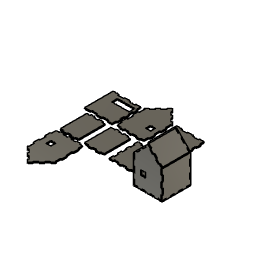
Verkefni2 v12 (Autodesk Fusion 360 design; units mm, degrees)
Autodesk Fusion 360 part; units mm, degrees
sketch "Botnplata Sketch" plane through (0, 0, 0) normal (0, 0, 1) x (1, 0, 0)
  line L0 (0, 0) -> (100, 0)
  line L1 (100, 0) -> (100, 100)
  line L2 (100, 100) -> (0, 100)
  line L3 (0, 100) -> (0, 0)
  dimension "d6" = 100
  dimension "d7" = 100
  constraint horizontal L0
  constraint vertical L1
  constraint horizontal L2
  constraint vertical L3
  constraint coincident L0.start L3.end
  measures "d6" distance of L0.start L2.end
  measures "d7" distance of L0.start L0.end
extrude "Extrude1" add sketch "Botnplata Sketch" along normal blind 4 makes body 1
sketch "Botnplatafingur Sketch" plane through (0, 0, 0) normal (0, -1, 0) x (1, 0, 0)
  line L0 (0, 0) -> (100, 0)
  line L1 (100, 0) -> (100, 4)
  line L2 (100, 4) -> (0, 4)
  line L3 (0, 4) -> (0, 0)
  line L4 (14.2857, 0) -> (28.5714, 0)
  line L5 (28.5714, 0) -> (28.5714, 4)
  line L6 (28.5714, 4) -> (14.2857, 4)
  line L7 (14.2857, 4) -> (14.2857, 0)
  dimension "d13" = 14.2857
  dimension "d14" = 14.2857
  constraint horizontal L4
  constraint vertical L5
  constraint horizontal L6
  constraint vertical L7
  constraint coincident L2 L5.end
  constraint coincident L0 L4.start
  measures "d13" distance of L5.end L6.end
  measures "d14" distance of L3 L7
extrude "Extrude2" cut sketch "Botnplatafingur Sketch" against normal blind 4 contours L0 L2 L4 L5 L6 L7 bodies 1
pattern_linear "R-Pattern1" count 3 spacing 28.5714 along (1, 0, 0) of "Extrude2"
sketch "Sketch3" plane through (100, 0, 0) normal (1, 0, 0) x (0, 1, 0)
  line L0 (0, 0) -> (100, 0)
  line L1 (100, 0) -> (100, 4)
  line L2 (100, 4) -> (0, 4)
  line L3 (0, 4) -> (0, 0)
  line L4 (14.2857, 0) -> (28.5714, 0)
  line L5 (28.5714, 0) -> (28.5714, 4)
  line L6 (28.5714, 4) -> (14.2857, 4)
  line L7 (14.2857, 4) -> (14.2857, 0)
  dimension "d21" = 14.2857
  dimension "d22" = 14.2857
  constraint horizontal L4
  constraint vertical L5
  constraint horizontal L6
  constraint vertical L7
  constraint coincident L2 L5.end
  constraint coincident L0 L4.start
  measures "d21" distance of L5.end L6.end
  measures "d22" distance of L3 L7
extrude "Extrude3" cut sketch "Sketch3" against normal blind 4 contours L0 L2 L4 L5 L6 L7 bodies 1
pattern_linear "R-Pattern2" count 3 spacing 28.5714 along (0, 1, 0) of "Extrude3"
sketch "Botnplafafingur Aftur Sketch" plane through (0, 0, 0) normal (-1, 0, 0) x (0, -1, 0)
  line L0 (-100, 0) -> (0, 0)
  line L1 (0, 0) -> (0, 4)
  line L2 (0, 4) -> (-100, 4)
  line L3 (-100, 4) -> (-100, 0)
  line L4 (-85.7143, 0) -> (-71.4286, 0)
  line L5 (-71.4286, 0) -> (-71.4286, 4)
  line L6 (-71.4286, 4) -> (-85.7143, 4)
  line L7 (-85.7143, 4) -> (-85.7143, 0)
  dimension "d29" = 14.2857
  dimension "d30" = 14.2857
  constraint horizontal L4
  constraint vertical L5
  constraint horizontal L6
  constraint vertical L7
  constraint coincident L2 L5.end
  constraint coincident L0 L4.start
  measures "d29" distance of L5.end L6.end
  measures "d30" distance of L3 L7
extrude "Extrude4" cut sketch "Botnplafafingur Aftur Sketch" against normal blind 4 contours L0 L2 L4 L5 L6 L7 bodies 1
pattern_linear "R-Pattern3" count 3 spacing 28.5714 along (0, -1, 0) of "Extrude4"
sketch "Sketch5" plane through (0, 100, 0) normal (0, 1, 0) x (-1, 0, 0)
  line L0 (-100, 0) -> (0, 0)
  line L1 (0, 0) -> (0, 4)
  line L2 (0, 4) -> (-100, 4)
  line L3 (-100, 4) -> (-100, 0)
  line L4 (-85.7143, 0) -> (-71.4286, 0)
  line L5 (-71.4286, 0) -> (-71.4286, 4)
  line L6 (-71.4286, 4) -> (-85.7143, 4)
  line L7 (-85.7143, 4) -> (-85.7143, 0)
  dimension "d37" = 14.2857
  dimension "d38" = 14.2857
  constraint horizontal L4
  constraint vertical L5
  constraint horizontal L6
  constraint vertical L7
  constraint coincident L2 L5.end
  constraint coincident L0 L4.start
  measures "d37" distance of L5.end L6.end
  measures "d38" distance of L3 L7
extrude "Extrude5" cut sketch "Sketch5" against normal blind 4 contours L0 L2 L4 L5 L6 L7 bodies 1
pattern_linear "R-Pattern4" count 3 spacing 28.5714 along (-1, 0, 0) of "Extrude5"
sketch "Sketch6" plane through (0, 0, 0) normal (1, 0, 0) x (0, 1, 0)
  line L0 (0, 0) -> (100, 0)
  line L1 (100, 0) -> (100, 100)
  line L2 (100, 100) -> (0, 100)
  line L3 (0, 100) -> (0, 0)
  dimension "d45" = 100
  dimension "d46" = 100
  constraint horizontal L0
  constraint vertical L1
  constraint horizontal L2
  constraint vertical L3
  constraint coincident L0.start L3.end
  measures "d45" distance of L0.start L2.end
  measures "d46" distance of L0.start L0.end
extrude "Extrude6" add sketch "Sketch6" along normal blind 4 separate body makes body 2
combine "Combine1" operation cut target body 2 tool bodies 1 keep tools
extrude "Extrude7" add 1 faces at (0, 47.619, 68) along direction (-1, 0, 0) blind 4 from surface at -100 separate body on bodies 2 makes body 3
sketch "Sketch9" plane through (0, 0, 0) normal (0, 1, 0) x (1, 0, 0)
  line L0 (0, 0) -> (0, -100)
  line L1 (0, -100) -> (50, -150)
  line L2 (50, -150) -> (100, -100)
  line L3 (100, -100) -> (100, 0)
  line L4 (100, 0) -> (0, 0)
  dimension "d66" = 135
  dimension "d67" = 135
  dimension "d68" = 100
  dimension "d69" = 100
  dimension "d70" = 100
  constraint coincident L0.start L4.end
  constraint vertical L0
  constraint parallel L0 L3
  constraint perpendicular L3 L4
  measures "d66" angle of L0 L1
  measures "d67" angle of L2 L3
  measures "d68" distance of L0.start L0.end
  measures "d69" distance of L2.end L3.end
  measures "d70" distance of L3.end L0.start
extrude "Extrude11" add sketch "Sketch9" along normal blind 4 separate body makes body 4
extrude "Extrude13" add 1 faces at (66.6667, 4, 66.6667) along direction (0, 1, 0) blind 4 from surface at 92 separate body on bodies 4 makes body 5
sketch "Sketch11" plane through (0, 100, 0) normal (0, 1, 0) x (-1, 0, 0)
  line L0 (0, 4) -> (0, 100)
  line L1 (0, 100) -> (-4, 100)
  line L2 (-4, 100) -> (-4, 4)
  line L3 (0, 80) -> (-4, 80)
  line L4 (-4, 80) -> (-4, 60)
  line L5 (-4, 60) -> (0, 60)
  line L6 (0, 60) -> (0, 80)
  line L7 (-4, 4) -> (0, 4)
  dimension "d90" = 20
  dimension "d91" = 20
  constraint horizontal L3
  constraint vertical L4
  constraint horizontal L5
  constraint vertical L6
  constraint coincident L2 L4.end
  constraint coincident L0 L3.start
  measures "d90" distance of L3.start L5.end
  measures "d91" distance of L1 L3
extrude "Extrude15" cut sketch "Sketch11" against normal blind 4 contours L0 L2 L3 L4 L5 L6 bodies 2
pattern_linear "R-Pattern5" count 2 spacing 40 along (0, 0, -1) of "Extrude15"
sketch "Sketch12" plane through (0, 100, 0) normal (0, 1, 0) x (-1, 0, 0)
  line L0 (-100, 100) -> (-100, 4)
  line L1 (-96, 4) -> (-96, 100)
  line L2 (-96, 100) -> (-100, 100)
  line L3 (-96, 80) -> (-100, 80)
  line L4 (-100, 80) -> (-100, 60)
  line L5 (-100, 60) -> (-96, 60)
  line L6 (-96, 60) -> (-96, 80)
  line L7 (-100, 4) -> (-96, 4)
  dimension "d98" = 20
  dimension "d99" = 20
  constraint horizontal L3
  constraint vertical L4
  constraint horizontal L5
  constraint vertical L6
  constraint coincident L0 L4.end
  constraint coincident L1 L3.start
  measures "d98" distance of L3.start L5.end
  measures "d99" distance of L2 L3
extrude "Extrude16" cut sketch "Sketch12" against normal blind 4 contours L0 L1 L3 L4 L5 L6 bodies 3
pattern_linear "R-Pattern6" count 2 spacing 40 along (0, 0, -1) of "Extrude16"
sketch "Sketch13" plane through (0, 0, 0) normal (0, -1, 0) x (1, 0, 0)
  line L0 (0, 4) -> (4, 4)
  line L1 (4, 4) -> (4, 100)
  line L2 (4, 100) -> (0, 100)
  line L3 (0, 100) -> (0, 4)
  line L4 (0, 80) -> (4, 80)
  line L5 (4, 80) -> (4, 60)
  line L6 (4, 60) -> (0, 60)
  line L7 (0, 60) -> (0, 80)
  dimension "d106" = 20
  dimension "d107" = 20
  constraint horizontal L4
  constraint vertical L5
  constraint horizontal L6
  constraint vertical L7
  constraint coincident L1 L5.end
  constraint coincident L3 L4.start
  measures "d106" distance of L2 L4
  measures "d107" distance of L4.start L6.end
extrude "Extrude17" cut sketch "Sketch13" against normal blind 4 contours L1 L3 L4 L5 L6 L7 bodies 2
pattern_linear "R-Pattern7" count 2 spacing 40 along (0, 0, -1) of "Extrude17"
sketch "Sketch14" plane through (0, 0, 0) normal (0, -1, 0) x (1, 0, 0)
  line L0 (100, 4) -> (100, 100)
  line L1 (100, 100) -> (96, 100)
  line L2 (96, 100) -> (96, 4)
  line L3 (96, 80) -> (100, 80)
  line L4 (100, 80) -> (100, 60)
  line L5 (100, 60) -> (96, 60)
  line L6 (96, 60) -> (96, 80)
  line L7 (96, 4) -> (100, 4)
  dimension "d114" = 20
  dimension "d115" = 20
  constraint horizontal L3
  constraint vertical L4
  constraint horizontal L5
  constraint vertical L6
  constraint coincident L0 L4.end
  constraint coincident L2 L3.start
  measures "d114" distance of L3.end L4.end
  measures "d115" distance of L1 L3
extrude "Extrude18" cut sketch "Sketch14" against normal blind 4 contours L0 L2 L3 L4 L5 L6 bodies 3
pattern_linear "R-Pattern8" count 2 spacing 40 along (0, 0, -1) of "Extrude18"
combine "Combine3" operation cut target body 4 tool bodies 2 1 3 keep tools
combine "Combine4" operation cut target body 5 tool bodies 2 1 3 keep tools
sketch "Sketch25" plane through (100, 0, 100) normal (0.707107, 0, 0.707107) x (0, 1, 0)
  line L0 (96, 0) -> (100, 0)
  line L1 (100, 0) -> (100, 70.7107)
  line L2 (100, 70.7107) -> (96, 70.7107)
  line L3 (100, 70.7107) -> (0, 70.7107)
  line L4 (0, 70.7107) -> (0, 3)
  line L5 (0, 3) -> (100, 3)
  line L6 (100, 3) -> (100, 70.7107)
  dimension "d123" = 100
  dimension "d136" = 67.7107
  constraint horizontal L3
  constraint vertical L4
  constraint horizontal L5
  constraint vertical L6
  constraint coincident L1.end L2.start
  measures "d123" distance of L4.end L5.end
  measures "d136" distance of L3.end L4.end
extrude "Extrude19" add sketch "Sketch25" against normal blind 4 separate body makes body 6
sketch "Sketch26" plane through (100, 0, 100) normal (0.707107, 0, 0.707107) x (0, 1, 0)
  line L0 (0, 70.7107) -> (0, 0)
  line L1 (0, 0) -> (4, 0)
  line L2 (4, 0) -> (4, 70.7107)
  line L3 (4, 70.7107) -> (0, 70.7107)
  line L4 (0, 56.5685) -> (4, 56.5685)
  line L5 (4, 56.5685) -> (4, 42.4264)
  line L6 (4, 42.4264) -> (0, 42.4264)
  line L7 (0, 42.4264) -> (0, 56.5685)
  dimension "d126" = 14.1421
  dimension "d127" = 14.1421
  constraint horizontal L4
  constraint vertical L5
  constraint horizontal L6
  constraint vertical L7
  constraint coincident L2 L5.end
  constraint coincident L0 L4.start
  measures "d126" distance of L4.end L5.end
  measures "d127" distance of L3 L4
extrude "Extrude20" cut sketch "Sketch26" against normal blind 4 contours L0 L2 L4 L5 L6 L7 bodies 4
pattern_linear "R-Pattern9" count 2 spacing 28.2843 along (0.707107, 0, -0.707107) of "Extrude20"
sketch "Sketch27" plane through (100, 0, 100) normal (0.707107, 0, 0.707107) x (0, 1, 0)
  line L0 (96, 70.7107) -> (96, 0)
  line L1 (96, 0) -> (100, 0)
  line L2 (100, 0) -> (100, 70.7107)
  line L3 (100, 70.7107) -> (96, 70.7107)
  line L4 (96, 56.5685) -> (100, 56.5685)
  line L5 (100, 56.5685) -> (100, 42.4264)
  line L6 (100, 42.4264) -> (96, 42.4264)
  line L7 (96, 42.4264) -> (96, 56.5685)
  dimension "d137" = 14.1421
  dimension "d138" = 14.1421
  constraint horizontal L4
  constraint vertical L5
  constraint horizontal L6
  constraint vertical L7
  constraint coincident L2 L5.end
  constraint coincident L0 L4.start
  measures "d137" distance of L4.end L5.end
  measures "d138" distance of L3 L4
extrude "Extrude21" cut sketch "Sketch27" against normal blind 4 contours L0 L2 L4 L5 L6 L7 bodies 5
pattern_linear "R-Pattern10" count 2 spacing 28.2843 along (0.707107, 0, -0.707107) of "Extrude21"
sketch "Sketch28" plane through (-50, 0, 50) normal (-0.707107, 0, 0.707107) x (0, -1, 0)
  line L0 (0, 70.7107) -> (0, 141.4214)
  line L1 (0, 141.4214) -> (-4, 141.4214)
  line L2 (-4, 141.4214) -> (-4, 70.7107)
  line L3 (-4, 70.7107) -> (0, 70.7107)
  line L4 (-4, 127.2792) -> (0, 127.2792)
  line L5 (0, 127.2792) -> (0, 113.1371)
  line L6 (0, 113.1371) -> (-4, 113.1371)
  line L7 (-4, 113.1371) -> (-4, 127.2792)
  dimension "d145" = 14.1421
  dimension "d146" = 14.1421
  constraint horizontal L4
  constraint vertical L5
  constraint horizontal L6
  constraint vertical L7
  constraint coincident L0 L5.end
  constraint coincident L2 L4.start
  measures "d145" distance of L4.end L5.end
  measures "d146" distance of L1 L4
extrude "Extrude22" cut sketch "Sketch28" against normal blind 4 contours L0 L2 L4 L5 L6 L7 bodies 4
pattern_linear "R-Pattern11" count 2 spacing 28.2843 along (-0.707107, 0, -0.707107) of "Extrude22"
sketch "Sketch29" plane through (-50, 0, 50) normal (-0.707107, 0, 0.707107) x (0, -1, 0)
  line L0 (-96, 70.7107) -> (-96, 141.4214)
  line L1 (-96, 141.4214) -> (-100, 141.4214)
  line L2 (-100, 141.4214) -> (-100, 70.7107)
  line L3 (-100, 70.7107) -> (-96, 70.7107)
  line L4 (-100, 127.2792) -> (-96, 127.2792)
  line L5 (-96, 127.2792) -> (-96, 113.1371)
  line L6 (-96, 113.1371) -> (-100, 113.1371)
  line L7 (-100, 113.1371) -> (-100, 127.2792)
  dimension "d153" = 14.1421
  dimension "d154" = 14.1421
  constraint horizontal L4
  constraint vertical L5
  constraint horizontal L6
  constraint vertical L7
  constraint coincident L0 L5.end
  constraint coincident L2 L4.start
  measures "d153" distance of L4.end L5.end
  measures "d154" distance of L1 L4
extrude "Extrude23" cut sketch "Sketch29" against normal blind 4 contours L0 L2 L4 L5 L6 L7 bodies 5
pattern_linear "R-Pattern12" count 2 spacing 28.2843 along (-0.707107, 0, -0.707107) of "Extrude23"
combine "Combine5" operation cut target body 6 tool bodies 5 4 keep tools
sketch "Sketch30" plane through (0, 100, 0) normal (0, 1, 0) x (-1, 0, 0)
  line L0 (-22.8284, 117.1716) -> (-20, 120)
  line L1 (-20, 120) -> (-30, 130)
  line L2 (-30, 130) -> (-32.8284, 127.1716)
  line L3 (-32.8284, 127.1716) -> (-42.8284, 137.1716)
  line L4 (-42.8284, 137.1716) -> (-40, 140)
  line L5 (-40, 140) -> (-50, 150)
  line L6 (-50, 150) -> (-60, 140)
  line L7 (-60, 140) -> (-57.1716, 137.1716)
  line L8 (-57.1716, 137.1716) -> (-67.1716, 127.1716)
  line L9 (-67.1716, 127.1716) -> (-70, 130)
  line L10 (-70, 130) -> (-80, 120)
  line L11 (-80, 120) -> (-77.1716, 117.1716)
  line L12 (-77.1716, 117.1716) -> (-87.1716, 107.1716)
  line L13 (-87.1716, 107.1716) -> (-90, 110)
  line L14 (-90, 110) -> (-100, 100)
  line L15 (-100, 100) -> (-96, 100)
  line L16 (-96, 100) -> (-96, 80)
  line L17 (-96, 80) -> (-100, 80)
  line L18 (-100, 80) -> (-100, 60)
  line L19 (-100, 60) -> (-96, 60)
  line L20 (-96, 60) -> (-96, 40)
  line L21 (-96, 40) -> (-100, 40)
  line L22 (-100, 40) -> (-100, 20)
  line L23 (-100, 20) -> (-96, 20)
  line L24 (-96, 20) -> (-96, 4)
  line L25 (-96, 4) -> (-85.7143, 4)
  line L26 (-85.7143, 4) -> (-85.7143, 0)
  line L27 (-85.7143, 0) -> (-71.4286, 0)
  line L28 (-71.4286, 0) -> (-71.4286, 4)
  line L29 (-71.4286, 4) -> (-57.1429, 4)
  line L30 (-57.1429, 4) -> (-57.1429, 0)
  line L31 (-57.1429, 0) -> (-42.8571, 0)
  line L32 (-42.8571, 0) -> (-42.8571, 4)
  line L33 (-42.8571, 4) -> (-28.5714, 4)
  line L34 (-28.5714, 4) -> (-28.5714, 0)
  line L35 (-28.5714, 0) -> (-14.2857, 0)
  line L36 (-14.2857, 0) -> (-14.2857, 4)
  line L37 (-14.2857, 4) -> (-4, 4)
  line L38 (-4, 4) -> (-4, 20)
  line L39 (-4, 20) -> (0, 20)
  line L40 (0, 20) -> (0, 40)
  line L41 (0, 40) -> (-4, 40)
  line L42 (-4, 40) -> (-4, 60)
  line L43 (-4, 60) -> (0, 60)
  line L44 (0, 60) -> (0, 80)
  line L45 (0, 80) -> (-4, 80)
  line L46 (-4, 80) -> (-4, 100)
  line L47 (-4, 100) -> (0, 100)
  line L48 (0, 100) -> (-10, 110)
  line L49 (-10, 110) -> (-12.8284, 107.1716)
  line L50 (-12.8284, 107.1716) -> (-22.8284, 117.1716)
  line L51 (-80, 60) -> (-63.3333, 60)
  line L52 (-63.3333, 60) -> (-63.3333, 43.3333)
  line L53 (-63.3333, 43.3333) -> (-80, 43.3333)
  line L54 (-80, 43.3333) -> (-80, 60)
  dimension "d165" = 16.6667
  dimension "d166" = 16.6667
  constraint horizontal L51
  constraint vertical L52
  constraint horizontal L53
  constraint vertical L54
  measures "d165" distance of L51.start L53.end
  measures "d166" distance of L51.start L51.end
extrude "Extrude24" cut sketch "Sketch30" against normal blind 4 contours L51 L52 L53 L54 bodies 5
sketch "Sketch31" plane through (0, 0, 0) normal (-1, 0, 0) x (0, -1, 0)
  line L0 (-4, 40) -> (0, 40)
  line L1 (0, 40) -> (0, 60)
  line L2 (0, 60) -> (-4, 60)
  line L3 (-4, 60) -> (-4, 80)
  line L4 (-4, 80) -> (0, 80)
  line L5 (0, 80) -> (0, 100)
  line L6 (0, 100) -> (-100, 100)
  line L7 (-100, 100) -> (-100, 80)
  line L8 (-100, 80) -> (-96, 80)
  line L9 (-96, 80) -> (-96, 60)
  line L10 (-96, 60) -> (-100, 60)
  line L11 (-100, 60) -> (-100, 40)
  line L12 (-100, 40) -> (-96, 40)
  line L13 (-96, 40) -> (-96, 20)
  line L14 (-96, 20) -> (-100, 20)
  line L15 (-100, 20) -> (-100, 4)
  line L16 (-100, 4) -> (-85.7143, 4)
  line L17 (-85.7143, 4) -> (-85.7143, 0)
  line L18 (-85.7143, 0) -> (-71.4286, 0)
  line L19 (-71.4286, 0) -> (-71.4286, 4)
  line L20 (-71.4286, 4) -> (-57.1429, 4)
  line L21 (-57.1429, 4) -> (-57.1429, 0)
  line L22 (-57.1429, 0) -> (-42.8571, 0)
  line L23 (-42.8571, 0) -> (-42.8571, 4)
  line L24 (-42.8571, 4) -> (-28.5714, 4)
  line L25 (-28.5714, 4) -> (-28.5714, 0)
  line L26 (-28.5714, 0) -> (-14.2857, 0)
  line L27 (-14.2857, 0) -> (-14.2857, 4)
  line L28 (-14.2857, 4) -> (0, 4)
  line L29 (0, 4) -> (0, 20)
  line L30 (0, 20) -> (-4, 20)
  line L31 (-4, 20) -> (-4, 40)
  line L32 (-85, 10) -> (-65, 10)
  line L33 (-65, 10) -> (-65, 70)
  line L34 (-65, 70) -> (-85, 70)
  line L35 (-85, 70) -> (-85, 10)
  dimension "d169" = 60
  dimension "d170" = 20
  constraint horizontal L32
  constraint vertical L33
  constraint horizontal L34
  constraint vertical L35
  measures "d169" distance of L32.start L34.end
  measures "d170" distance of L32.start L32.end
extrude "Extrude25" cut sketch "Sketch31" against normal blind 4 contours L32 L33 L34 L35 bodies 2
sketch "Sketch32" plane through (0, 0, 0) normal (0, -1, 0) x (1, 0, 0)
  line L0 (20, 120) -> (22.8284, 117.1716)
  line L1 (22.8284, 117.1716) -> (12.8284, 107.1716)
  line L2 (12.8284, 107.1716) -> (10, 110)
  line L3 (10, 110) -> (0, 100)
  line L4 (0, 100) -> (4, 100)
  line L5 (4, 100) -> (4, 80)
  line L6 (4, 80) -> (0, 80)
  line L7 (0, 80) -> (0, 60)
  line L8 (0, 60) -> (4, 60)
  line L9 (4, 60) -> (4, 40)
  line L10 (4, 40) -> (0, 40)
  line L11 (0, 40) -> (0, 20)
  line L12 (0, 20) -> (4, 20)
  line L13 (4, 20) -> (4, 4)
  line L14 (4, 4) -> (14.2857, 4)
  line L15 (14.2857, 4) -> (14.2857, 0)
  line L16 (14.2857, 0) -> (28.5714, 0)
  line L17 (28.5714, 0) -> (28.5714, 4)
  line L18 (28.5714, 4) -> (42.8571, 4)
  line L19 (42.8571, 4) -> (42.8571, 0)
  line L20 (42.8571, 0) -> (57.1429, 0)
  line L21 (57.1429, 0) -> (57.1429, 4)
  line L22 (57.1429, 4) -> (71.4286, 4)
  line L23 (71.4286, 4) -> (71.4286, 0)
  line L24 (71.4286, 0) -> (85.7143, 0)
  line L25 (85.7143, 0) -> (85.7143, 4)
  line L26 (85.7143, 4) -> (96, 4)
  line L27 (96, 4) -> (96, 20)
  line L28 (96, 20) -> (100, 20)
  line L29 (100, 20) -> (100, 40)
  line L30 (100, 40) -> (96, 40)
  line L31 (96, 40) -> (96, 60)
  line L32 (96, 60) -> (100, 60)
  line L33 (100, 60) -> (100, 80)
  line L34 (100, 80) -> (96, 80)
  line L35 (96, 80) -> (96, 100)
  line L36 (96, 100) -> (100, 100)
  line L37 (100, 100) -> (90, 110)
  line L38 (90, 110) -> (87.1716, 107.1716)
  line L39 (87.1716, 107.1716) -> (77.1716, 117.1716)
  line L40 (77.1716, 117.1716) -> (80, 120)
  line L41 (80, 120) -> (70, 130)
  line L42 (70, 130) -> (67.1716, 127.1716)
  line L43 (67.1716, 127.1716) -> (57.1716, 137.1716)
  line L44 (57.1716, 137.1716) -> (60, 140)
  line L45 (60, 140) -> (50, 150)
  line L46 (50, 150) -> (40, 140)
  line L47 (40, 140) -> (42.8284, 137.1716)
  line L48 (42.8284, 137.1716) -> (32.8284, 127.1716)
  line L49 (32.8284, 127.1716) -> (30, 130)
  line L50 (30, 130) -> (20, 120)
  line L51 (41.6667, 43.333) -> (25, 43.333)
  line L52 (25, 43.333) -> (25, 59.9997)
  line L53 (25, 59.9997) -> (41.6667, 59.9997)
  line L54 (41.6667, 59.9997) -> (41.6667, 43.333)
  dimension "d174" = 16.6667
  dimension "d175" = 16.6667
  constraint horizontal L51
  constraint vertical L52
  constraint horizontal L53
  constraint vertical L54
  measures "d174" distance of L52.end L53.end
  measures "d175" distance of L51.start L53.end
extrude "Extrude26" cut sketch "Sketch32" against normal blind 4 contours L51 L52 L53 L54 bodies 4
sketch "Sketch34" plane through (-50, 0, 50) normal (-0.707107, 0, 0.707107) x (0, -1, 0)
  line L0 (-100, 98.9949) -> (-96, 98.9949)
  line L1 (-96, 98.9949) -> (-96, 113.1371)
  line L2 (-96, 113.1371) -> (-100, 113.1371)
  line L3 (-100, 113.1371) -> (-100, 98.9949)
combine "Combine7" operation cut target body 6 tool bodies 3 keep tools
sketch "Sketch38" plane through (-50, 0, 50) normal (-0.707107, 0, 0.707107) x (0, -1, 0)
  line L0 (-100, 137.4) -> (0, 137.4)
  line L1 (0, 137.4) -> (0, 73.6893)
  line L2 (0, 73.6893) -> (-100, 73.6893)
  line L3 (-100, 73.6893) -> (-100, 137.4)
  dimension "d188" = 100
  dimension "d189" = 63.7107
  constraint horizontal L0
  constraint vertical L1
  constraint horizontal L2
  constraint vertical L3
  measures "d188" distance of L0.start L0.end
  measures "d189" distance of L0.start L2.end
extrude "Extrude29" add sketch "Sketch38" against normal blind 4 separate body makes body 7
combine "Combine8" operation cut target body 7 tool bodies 4 5 keep tools
copy_body "CopyPasteBodies1" bodies 1 7 6 2 4 3 5 makes body 8 makes body 9 makes body 10 makes body 11 makes body 12 makes body 13 makes body 14 in component "Camlay"
move_body "Move1" bodies 8 9 10 11 12 13 14 to x (1, 0, 0) y (0, 1, 0) z (0, 0, 1) at (-210.9779, 36.1473, 0) in component "Camlay"
move_body "Align1" bodies 13 to x (0, 0, 1) y (0, 1, 0) z (-1, 0, 0) at (-60.9779, 0, 114.9779) in component "Camlay"
move_body "Align2" bodies 14 to x (1, 0, 0) y (0, 0, -1) z (0, 1, 0) at (0, 57.1473, 136.1473) in component "Camlay"
move_body "Align3" bodies 10 to x (0.707107, 0, 0.707107) y (0, 1, 0) z (-0.707107, 0, 0.707107) at (49.0007, 0, 11.7626) in component "Camlay"
move_body "Align4" bodies 11 to x (0, 0, 1) y (0, 1, 0) z (-1, 0, 0) at (-156.9779, 0, 210.9779) in component "Camlay"
move_body "Align5" bodies 9 to x (0.707107, 0, -0.707107) y (0, 1, 0) z (0.707107, 0, 0.707107) at (-139.8789, 0, -211.8946) in component "Camlay"
move_body "Align6" bodies 9 to x (1, 0, 0) y (0, 1, 0) z (0, 0, 1) at (0, 0, -4) in component "Camlay"
move_body "Move2" bodies 14 to x (1, 0, 0) y (0, 1, 0) z (0, 0, 1) at (0, 90, 0) in component "Camlay"
move_body "Move3" bodies 11 to x (1, 0, 0) y (0, 1, 0) z (0, 0, 1) at (-59.6927, 109.6715, 0) in component "Camlay"
move_body "Move4" bodies 13 to x (1, 0, 0) y (0, 1, 0) z (0, 0, 1) at (59.6927, 115.4437, 0) in component "Camlay"
move_body "Move5" bodies 8 to x (1, 0, 0) y (0, 1, 0) z (0, 0, 1) at (140, 0, 0) in component "Camlay"
move_body "Move6" bodies 9 to x (1, 0, 0) y (0, 1, 0) z (0, 0, 1) at (-80, 0, 0) in component "Camlay"
move_body "Move7" bodies 10 to x (1, 0, 0) y (0, 1, 0) z (0, 0, 1) at (-40, 0, 0) in component "Camlay"
move_body "Move8" bodies 8 to x (1, 0, 0) y (0, 1, 0) z (0, 0, 1) at (-50, 0, 0) in component "Camlay"
move_body "Align7" bodies 12 to x (1, 0, 0) y (0, 0, 1) z (0, -1, 0) at (0, 111.1473, -32.1473) in component "Camlay"
move_body "Align8" bodies 12 to x (1, 0, 0) y (0, 1, 0) z (0, 0, 1) at (0, 0, -4) in component "Camlay"
move_body "Move9" bodies 12 to x (1, 0, 0) y (0, 1, 0) z (0, 0, 1) at (-90, -80, 0) in component "Camlay"
component "Camlay" placed x (1, 0, 0) y (0, 1, 0) z (0, 0, 1) at (0, 0, 0)
equation "Botnlengd = 100 mm"
equation "Botnbreidd = 100 mm"
equation "Þykkt = 4 mm"
equation "Hæð = 100 mm"
equation "Þakhalli = 45 deg"
equation "d6 = Botnbreidd"
equation "d7 = Botnlengd"
equation "d8 = Þykkt"
equation "Botnfingur = 3"
equation "Þakfingur = 2"
equation "Fingurbreiddbotn = Botnlengd / ( ( Botnfingur * 2 ) + 1 )"
equation "d13 = Fingurbreiddbotn"
equation "d14 = Fingurbreiddbotn"
equation "d15 = -Þykkt"
equation "d17 = Botnfingur"
equation "d19 = Botnlengd - ( Fingurbreiddbotn * 3 )"
equation "d21 = Fingurbreiddbotn"
equation "d22 = Fingurbreiddbotn"
equation "d23 = -Þykkt"
equation "d25 = Botnfingur"
equation "d27 = -( Botnlengd - Fingurbreiddbotn * 3 )"
equation "d29 = Fingurbreiddbotn"
equation "d30 = Fingurbreiddbotn"
equation "d31 = -Þykkt"
equation "d33 = Botnfingur"
equation "d35 = Botnlengd - ( Fingurbreiddbotn * 3 )"
equation "d37 = Fingurbreiddbotn"
equation "d38 = Fingurbreiddbotn"
equation "d39 = -Þykkt"
equation "d41 = Botnfingur"
equation "d43 = Botnlengd - ( Fingurbreiddbotn * 3 )"
equation "d45 = Hæð"
equation "d46 = Botnlengd"
equation "d47 = Þykkt"
equation "d50 = -Botnlengd"
equation "d51 = Þykkt"
equation "d66 = 90 deg + Þakhalli"
equation "d67 = 90 deg + Þakhalli"
equation "d68 = Hæð"
equation "d69 = Hæð"
equation "d70 = Botnlengd"
equation "d76 = Þykkt"
equation "d81 = Þykkt - Botnlengd"
equation "d82 = Þykkt"
equation "Hliðarfingur = 2"
equation "FingurbreiddHlið = Hæð / ( ( Hliðarfingur * 2 + 1 ) )"
equation "d90 = FingurbreiddHlið"
equation "d91 = FingurbreiddHlið"
equation "d92 = -Þykkt"
equation "d94 = Hliðarfingur"
equation "d96 = -( Hæð - ( FingurbreiddHlið * 3 ) )"
equation "d98 = FingurbreiddHlið"
equation "d99 = FingurbreiddHlið"
equation "d100 = -Þykkt"
equation "d102 = Hliðarfingur"
equation "d104 = -( Hæð - ( FingurbreiddHlið * 3 ) )"
equation "d106 = FingurbreiddHlið"
equation "d107 = FingurbreiddHlið"
equation "d108 = -Þykkt"
equation "d110 = Hliðarfingur"
equation "d112 = ( Hæð - ( FingurbreiddHlið * 3 ) )"
equation "d114 = FingurbreiddHlið"
equation "d115 = FingurbreiddHlið"
equation "d116 = -Þykkt"
equation "d118 = Hliðarfingur"
equation "d120 = -( Hæð - ( FingurbreiddHlið * 3 ) )"
equation "d123 = Botnlengd"
equation "d124 = -Þykkt"
equation "d126 = Fingurbreiddþak"
equation "d127 = Fingurbreiddþak"
equation "d128 = -Þykkt"
equation "Þakpar1 = 50" comment "Helmingur af Botnlengd"
equation "Þakplatalengd = ( sqrt(2 * ( Þakpar1 * Þakpar1 )) ) * 1 mm"
equation "d132 = Þakfingur"
equation "d134 = -( Þakplatalengd - ( Fingurbreiddþak * 3 ) )"
equation "d136 = Þakplatalengd - 3 mm"
equation "d137 = Fingurbreiddþak"
equation "d138 = Fingurbreiddþak"
equation "d139 = -Þykkt"
equation "d141 = Þakfingur"
equation "d143 = ( Þakplatalengd - ( Fingurbreiddþak * 3 ) )"
equation "d145 = Fingurbreiddþak"
equation "d146 = Fingurbreiddþak"
equation "d147 = -Þykkt"
equation "d149 = Þakfingur"
equation "d151 = ( Þakplatalengd - ( Fingurbreiddþak * 3 ) )"
equation "d153 = Fingurbreiddþak"
equation "d154 = Fingurbreiddþak"
equation "d155 = -Þykkt"
equation "d157 = Þakfingur"
equation "d159 = -( Þakplatalengd - ( Fingurbreiddþak * 3 ) )"
equation "Fingurbreiddþak = Þakplatalengd / ( ( Þakfingur * 2 ) + 1 )"
equation "gluggi = Botnlengd / 6"
equation "hurðbotn = Botnlengd / 5"
equation "hurðhæð = Hæð * 0.6"
equation "d165 = gluggi"
equation "d166 = gluggi"
equation "d167 = -Þykkt"
equation "d169 = hurðhæð"
equation "d170 = hurðbotn"
equation "d171 = -Þykkt"
equation "d174 = gluggi"
equation "d175 = gluggi"
equation "d176 = -Þykkt"
equation "d188 = Botnlengd"
equation "d189 = Þakplatalengd - 7 mm"
equation "d190 = -Þykkt"
named bodies: "Botnplata", "Framhlið", "Bakhlið", "HHlið", "VHlið", "Þakplatabak", "Þakplatafram"
